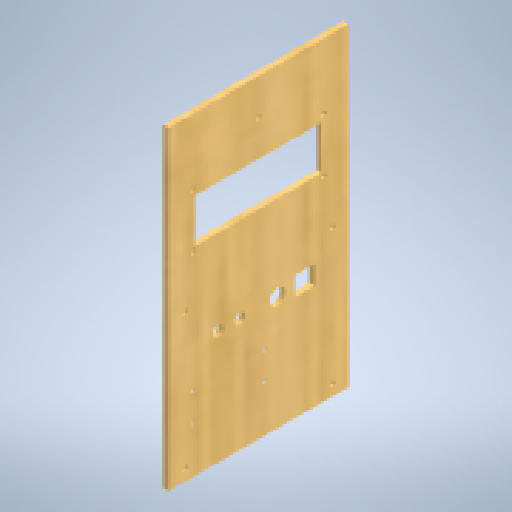
# Autodesk Inventor part: Panel1
Saved by Autodesk Inventor 2023 (Build 270158000, 158)
## iProperties
Created: 2022-12-03
Part Number: Panel1
Material: Genérico
Document SubType Name: Modeling
Designer: sergi
Density: 1 g/cm^3
Appearance: Valor por defecto
Author: sergi
Autodesk Inventor part; units mm, degrees
ref_plane "YZ Plane" through (0, 0, 0) normal (1, 0, 0) x (0, 1, 0)
ref_plane "XZ Plane" through (0, 0, 0) normal (0, 1, 0) x (-1, 0, 0)
ref_plane "XY Plane" through (0, 0, 0) normal (0, 0, 1) x (1, 0, 0)
sketch "Boceto1" plane through (0, 0, 0) normal (0, 1, 0) x (-1, 0, 0)
  line L0 (-1.5, -51.5) -> (1.5, -51.5)
  line L1 (1.5, -51.5) -> (1.5, 51.5)
  line L2 (1.5, 51.5) -> (-1.5, 51.5)
  line L3 (-1.5, 51.5) -> (-1.5, -51.5)
  line L4 (-1.5, -51.5) -> (1.5, 51.5) construction
  line L5 (1.5, -51.5) -> (-1.5, 51.5) construction
  point P0 (0, 0)
  dimension "d0" = 3
  dimension "d1" = 103
  constraints: 12 end point, 2 midpoint, 2 parallel, 1 horizontal, 1 perpendicular
  measures "d0" distance of L2.end L1.end
  measures "d1" distance of L1.end L0.end
extrude "Extrusión1" add sketch "Boceto1" along normal blind 180
sketch "Boceto2" plane through (-1.5, 0, -51.5) normal (-1, 0, 0) x (0, 0, 1)
  line L0 (3, 148.5) -> (100, 148.5) projected
  line L1 (9.3714, 170) -> (39, 160.0424) projected
  line L2 (9.3714, 170) -> (93.6286, 170) projected
  line L3 (51.5, 148.5) -> (51.5, 170)
  circle A0 centre (51.5, 159.25) radius 1.5
  circle A1 centre (93.5, 84) radius 1.5 projected
  circle A2 centre (9.5, 84) radius 1.5 projected
  circle A3 centre (93.5, 6.5) radius 1.25 projected
  circle A4 centre (9.5, 6.5) radius 1.25 projected
  line L4 (3, 0) -> (16, 0) projected
  line L5 (16, 0) -> (16, 13) projected
  line L6 (3, 13) -> (16, 13) projected
  line L7 (3, 0) -> (3, 13) projected
  circle A5 centre (9.5, 6.5) radius 1.25 projected
  point P0 (51.5, 0)
  dimension "d4" = 3
  constraints: 3 midpoint, 2 end point, 1 centre point
  measures "d4" diameter of A0
hole "Agujero1" at (-1.5, 159.25, 0) at (-1.5, 6.5, -42) at (-1.5, 84, -42) at (-1.5, 84, 42) at (-1.5, 6.5, 42) direction (1, 0, 0) diameter 3 depth 5 tip angle 118
sketch "Boceto3" plane through (-1.5, 0, -51.5) normal (-1, 0, 0) x (0, 0, 1)
  circle A0 centre (13.05, 20.58) radius 3.1754 projected
  circle A1 centre (13.05, 47.42) radius 3.1754 projected
  circle A2 centre (42.45, 20.58) radius 3.1754 projected
  circle A3 centre (42.45, 47.42) radius 3.1754 projected
  line L0 (20.6, 69.9) -> (29.6, 69.9) projected
  line L1 (20.6, 69.9) -> (20.6, 60.9) projected
  line L2 (20.6, 60.9) -> (29.6, 60.9) projected
  line L3 (29.6, 60.9) -> (29.6, 69.9) projected
  circle A4 centre (40.5996, 65.0004) radius 3.4994 projected
  circle A5 centre (62.1002, 64.9998) radius 2.0003 projected
  circle A6 centre (74.6001, 65) radius 2.0001 projected
  circle A7 centre (53, 27) radius 0.75 projected
  circle A8 centre (55.5, 43) radius 1 projected
  circle A9 centre (91.5, 27) radius 1 projected
  circle A10 centre (94.0001, 27) radius 0.7499 projected
  circle A11 centre (93.9999, 43.0001) radius 0.7499 projected
  circle A12 centre (89.575, 56.025) radius 1.0751 projected
  circle A13 centre (89.5749, 71.975) radius 1.0749 projected
  circle A14 centre (13.6251, 71.975) radius 1.0751 projected
  circle A15 centre (13.625, 56.0251) radius 1.0749 projected
  circle A16 centre (53, 43) radius 0.75 projected
  line L4 (30.1, 70.4) -> (20.1, 70.4)
  line L5 (20.1, 70.4) -> (20.1, 60.4)
  line L6 (20.1, 60.4) -> (30.1, 60.4)
  line L7 (30.1, 60.4) -> (30.1, 70.4)
  circle A17 centre (40.5996, 65.0004) radius 4.4994
  circle A18 centre (62.1002, 64.9998) radius 3.0003
  circle A19 centre (74.6001, 65) radius 3.0001
  line L8 (19.6, 59.9) -> (19.6, 70.9)
  line L9 (19.6, 70.9) -> (30.6, 70.9)
  line L10 (30.6, 70.9) -> (30.6, 59.9)
  line L11 (30.6, 59.9) -> (19.6, 59.9)
  line L12 (15.85, 138.4) -> (15.85, 114.4) projected
  line L13 (87.15, 138.4) -> (15.85, 138.4) projected
  line L14 (15.85, 114.4) -> (87.15, 114.4) projected
  line L15 (87.15, 114.4) -> (87.15, 138.4) projected
  circle A20 centre (14.15, 142.45) radius 1.45 projected
  circle A21 centre (14.15, 111.55) radius 1.45 projected
  circle A22 centre (89.05, 111.55) radius 1.45 projected
  circle A23 centre (89.05, 142.45) radius 1.45 projected
  line L16 (15.35, 138.9) -> (15.35, 113.9)
  line L17 (15.35, 113.9) -> (87.65, 113.9)
  line L18 (87.65, 113.9) -> (87.65, 138.9)
  line L19 (87.65, 138.9) -> (15.35, 138.9)
  circle A24 centre (42.45, 47.42) radius 1.5
  circle A25 centre (13.05, 47.42) radius 1.5
  circle A26 centre (13.05, 20.58) radius 1.5
  circle A27 centre (42.45, 20.58) radius 1.5
  circle A28 centre (14.15, 111.55) radius 1.5
  point P0 (51.5, 0)
  dimension "d12" = 0.5
  dimension "d13" = 1
  dimension "d14" = 1
  dimension "d15" = 1
  dimension "d16" = 0.5
  dimension "d17" = 0.5
  dimension "d18" = 3
  dimension "d19" = 3
  dimension "d20" = 3
  dimension "d21" = 3
  dimension "d22" = 3
  constraints: 24 end point, 8 centre point, 5 coincident, 9 other
  measures "d12" distance between parallel lines of L0 L4
  measures "d13" radial gap between concentric circles of A4 A17
  measures "d14" radial gap between concentric circles of A5 A18
  measures "d15" radial gap between concentric circles of A6 A19
  measures "d16" distance between parallel lines of L5 L8
  measures "d17" distance between parallel lines of L13 L19
  measures "d18" diameter of A24
  measures "d19" diameter of A25
  measures "d20" diameter of A26
  measures "d21" diameter of A27
  measures "d22" diameter of A28
extrude "Extrusión2" cut sketch "Boceto3" against normal through all contours L0 L3 L2 L1 | A4 | A5 | A6 | L7 L6 L5 L4 | A17 | A18 | A19 | L8 L9 L10 L11 | L13 L15 L14 L12 | A20 | A21 | A22 | A23 | L19 L18 L17 L16
hole "Agujero2" at (-1.5, 43, -3.5) at (-1.5, 27.0001, -3.5001) at (-1.5, 27, 37.5) at (-1.5, 43, 37.5) direction (1, 0, 0) diameter 2 end through all
sketch "Boceto5" plane through (-1.5, 0, -51.5) normal (-1, 0, 0) x (0, 0, 1)
  circle A0 centre (21.1, 22.5) radius 1.5 projected
  circle A1 centre (21.1, 40.95) radius 1.5 projected
  circle A2 centre (34.5, 40.95) radius 1.5 projected
  circle A3 centre (34.5, 22.5) radius 1.5 projected
  point P0 (51.5, 0)
hole "Agujero3" at (-1.5, 40.95, -17) at (-1.5, 40.95, -30.4) at (-1.5, 22.5, -30.4) at (-1.5, 22.5, -17) direction (1, 0, 0) diameter 3 end through all
